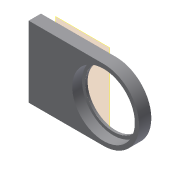
# Autodesk Inventor part: 10_Filteslide_25mm
Saved by Autodesk Inventor 2019 (Build 230136000, 136)
## iProperties
Created: 2019-08-26
Part Number: 10_Filteslide_25mm
Material: Generic
Document SubType Name: Modeling
Designer: diederichbenedict
Density: 1 g/cm^3
Appearance: Default
Author: diederichbenedict
Autodesk Inventor part; units mm, degrees
ref_plane "YZ Plane" through (0, 0, 0) normal (1, 0, 0) x (0, 1, 0)
ref_plane "XZ Plane" through (0, 0, 0) normal (0, 1, 0) x (-1, 0, 0)
ref_plane "XY Plane" through (0, 0, 0) normal (0, 0, 1) x (1, 0, 0)
ref_plane "Work Plane1" through (0, 0, 0) normal (0, 0, 1) x (1, 0, 0)
sketch "Sketch1" plane through (0, 0, 0) normal (0, 0, 1) x (1, 0, 0)
  arc A0 (-18.155, 30) -> (-18.155, 0) centre (0, 15) ccw construction
  line L0 (-18.155, 0) -> (-3.4871, 0) construction
  arc A1 (-3.4871, 30) -> (-3.4871, 0) centre (0, 15) ccw construction
  line L1 (-18.155, 30) -> (-3.4871, 30) construction
  circle A2 centre (0, 15) radius 15.4 construction
  arc A3 (-6.5238, 29.5) -> (-6.5238, 0.5) centre (0, 15) ccw construction
  line L2 (-6.5238, 0.5) -> (-17.9179, 0.5) construction
  arc A4 (-17.9179, 29.5) -> (-17.9179, 0.5) centre (0, 15) ccw construction
  line L3 (-17.9179, 29.5) -> (-6.5238, 29.5) construction
  circle A5 centre (0, 15) radius 12.775 construction
  line L4 (-6.5238, 29.5) -> (0, 29.5) construction
  line L5 (-6.5238, 0.5) -> (0, 0.5) construction
  arc A6 (0, 0.5) -> (0, 29.5) centre (0, 15) ccw construction
  line L6 (-42.0841, 29.5) -> (-42.0841, 0.5)
  line L7 (-42.0841, 0.5) -> (0, 0.5)
  line L8 (-42.0841, 29.5) -> (0, 29.5)
  circle A7 centre (0, 15) radius 11.5
  arc A8 (0, 0.5) -> (0, 29.5) centre (0, 15) ccw
  point P0 (0, 0)
  dimension "d0" = 0.5
  dimension "d1" = 25.55
  dimension "d2" = 23
  constraints: 14 end point, 8 point on circle, 6 centre point, 3 tangent, 2 coincident, 2 point on line, 1 parallel, 1 perpendicular, 1 vertical, 3 other
  measures "d0" distance between parallel lines of L1 L3
  measures "d1" diameter of A5
  measures "d2" diameter of A7
extrude "Extrusion1" add sketch "Sketch1" along normal blind 1
sketch "Sketch2" plane through (0, 0, 1) normal (0, 0, 1) x (1, 0, 0)
  circle A0 centre (0, 15) radius 11.5 projected
  line L0 (0, 29.5) -> (-42.0841, 29.5) projected
  line L1 (-42.0841, 29.5) -> (-42.0841, 0.5) projected
  line L2 (-42.0841, 0.5) -> (0, 0.5) projected
  arc A1 (0, 0.5) -> (0, 29.5) centre (0, 15) ccw projected
  circle A2 centre (0, 15) radius 12.775
  point P0 (0, 0)
  dimension "d5" = 25.55
  constraints: 1 centre point, 1 coincident
  measures "d5" diameter of A2
extrude "Extrusion2" add sketch "Sketch2" along normal blind 4 contours A1 L2 L1 L0
body "Solid1"
